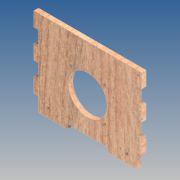
# Autodesk Inventor part: 2204_Housing Front_V1
Saved by Autodesk Inventor 2020 (Build 240168000, 168)
## iProperties
Created: 2019-11-08
Part Number: 2204_Housing Front_V1
Material: Wood (Birch)
Document SubType Name: Modeling
Designer: RFLab
Density: 0.55 g/cm^3
Appearance: Birch - Natural Polished
Author: RFLab
Autodesk Inventor part; units mm, degrees
ref_plane "YZ Plane" through (0, 0, 0) normal (1, 0, 0) x (0, 1, 0)
ref_plane "XZ Plane" through (0, 0, 0) normal (0, 1, 0) x (-1, 0, 0)
ref_plane "XY Plane" through (0, 0, 0) normal (0, 0, 1) x (1, 0, 0)
sketch "Sketch1" plane through (0, 0, 0) normal (0, 0, 1) x (1, 0, 0)
  line L0 (-75, 60) -> (75, 60)
  line L1 (75, 60) -> (75, -60)
  line L2 (75, -60) -> (-75, -60)
  line L3 (-75, -60) -> (-75, 60)
  point P0 (0, 0)
  dimension "d0" = 150
  dimension "d1" = 120
  dimension "d2" = 60
  dimension "d3" = 75
  constraints: 8 end point, 2 parallel, 1 horizontal, 1 perpendicular
  measures "d0" distance of L1.end L2.end
  measures "d1" distance of L0.end L1.end
  measures "d2" distance from line of point (0, 0) L2
  measures "d3" distance from line of L3 point (0, 0)
extrude "Extrusion1" add sketch "Sketch1" along normal blind 6.35
sketch "Sketch2" plane through (0, 0, 6.35) normal (0, 0, 1) x (1, 0, 0)
  line L0 (-75, 60) -> (-75, -60) projected
  line L1 (-75, 40) -> (-68.65, 40)
  line L2 (-68.65, 40) -> (-68.65, 20)
  line L3 (-68.65, 20) -> (-75, 20)
  line L4 (-75, 20) -> (-75, 40)
  line L5 (-75, 60) -> (-75, -60) projected
  line L6 (-75, 0) -> (-68.65, 0)
  line L7 (-68.65, 0) -> (-68.65, -20)
  line L8 (-68.65, -20) -> (-75, -20)
  line L9 (-75, -20) -> (-75, 0)
  line L10 (-75, -40) -> (-68.65, -40)
  line L11 (-68.65, -40) -> (-68.65, -60)
  line L12 (-68.65, -60) -> (-75, -60)
  line L13 (-75, -60) -> (-75, -40)
  line L14 (75, -60) -> (75, 60) projected
  line L15 (75, 40) -> (68.65, 40)
  line L16 (68.65, 40) -> (68.65, 20)
  line L17 (68.65, 20) -> (75, 20)
  line L18 (75, 20) -> (75, 40)
  line L19 (75, 0) -> (68.65, 0)
  line L20 (68.65, 0) -> (68.65, -20)
  line L21 (68.65, -20) -> (75, -20)
  line L22 (75, -20) -> (75, 0)
  line L23 (75, -40) -> (68.65, -40)
  line L24 (68.65, -40) -> (68.65, -60)
  line L25 (68.65, -60) -> (75, -60)
  line L26 (75, -60) -> (75, -40)
  line L27 (-75, -60) -> (75, -60) projected
  line L28 (-28.65, -60) -> (28.65, -60)
  line L29 (28.65, -60) -> (28.65, -53.65)
  line L30 (28.65, -53.65) -> (-28.65, -53.65)
  line L31 (-28.65, -53.65) -> (-28.65, -60)
  line L32 (75, 60) -> (-75, 60) projected
  line L33 (-28.65, 60) -> (28.65, 60)
  point P0 (0, 0)
  dimension "d6" = 6.35
  dimension "d7" = 20
  dimension "d8" = 20
  dimension "d9" = 20
  dimension "d10" = 20
  dimension "d11" = 20
  dimension "d12" = 20
  dimension "d13" = 20
  dimension "d22" = 57.3
  dimension "d23" = 46.35
  dimension "d24" = 46.35
  dimension "d26" = 6.35
  constraints: 58 end point, 14 parallel, 9 point on line, 8 horizontal, 7 equal length, 7 perpendicular, 2 midpoint
  measures "d6" distance of L1.start L1.end
  measures "d7" distance of L1.end L2.end
  measures "d8" distance of L1.start L0.start
  measures "d9" distance of L6.start L3.end
  measures "d10" distance of L10.start L8.end
  measures "d11" distance of L15.start L14.end
  measures "d12" distance of L19.start L17.end
  measures "d13" distance of L23.start L21.end
  measures "d22" distance of L29.end L30.end
  measures "d23" distance of L14.start L28.end
  measures "d24" distance of L14.end L33.end
  measures "d26" distance of L30.end L28.start
extrude "Extrusion2" cut sketch "Sketch2" against normal through all contours L1 L2 L3 L0 | L6 L7 L8 L0 | L14 L17 L16 L15 | L10 L11 L12 L0 | L14 L21 L20 L19 | L31 L30 L29 L27 | L14 L25 L24 L23
sketch "Sketch3" plane through (0, 0, 6.35) normal (0, 0, 1) x (1, 0, 0)
  circle A0 centre (0, -4.5) radius 27
  line L0 (-75, -60) -> (75, -60) projected
  line L1 (75, 40) -> (75, 60) projected
  point P0 (0, 0)
  dimension "d16" = 55.5
  dimension "d17" = 75
  dimension "d18" = 54
  constraints: 1 centre point
  measures "d16" distance from line of L0 A0.centre
  measures "d17" distance from line of L1 A0.centre
  measures "d18" diameter of A0
extrude "Extrusion3" cut sketch "Sketch3" against normal through all
sketch "Sketch4" plane through (0, 0, 6.35) normal (0, 0, 1) x (1, 0, 0)
  circle A0 centre (0, -4.5) radius 27 projected
  circle A1 centre (0, -4.5) radius 33.5
  circle A2 centre (23.6881, 19.1881) radius 1.75
  line L0 (0, -4.5) -> (33.5, -4.5)
  line L1 (0, -4.5) -> (23.6881, 19.1881)
  point P0 (0, 0)
  dimension "d27" = 67
  dimension "d28" = 45
  dimension "d29" = 3.5
  constraints: 4 end point, 2 centre point, 2 point on circle, 1 coincident, 1 horizontal
  measures "d27" diameter of A1
  measures "d28" angle of L1 L0
  measures "d29" diameter of A2
extrude "Extrusion4" cut sketch "Sketch4" against normal through all contours L1 A1 A2 | A2 A1 L1 | A1 A2
pattern_circular "Circular Pattern1" count 4 over 360 about axis through (0, -4.5, 6.35) along (0, 0, -1) of "Extrusion4"
sketch "Sketch5" plane through (0, 0, 6.35) normal (0, 0, 1) x (1, 0, 0)
  circle A0 centre (-54.9, -48) radius 1.75
  circle A1 centre (54.9, -48) radius 1.75
  line L0 (-68.65, -60) -> (-28.65, -60) projected
  line L1 (-75, -20) -> (-75, -40) projected
  line L2 (75, -40) -> (75, -20) projected
  line L3 (28.65, -60) -> (68.65, -60) projected
  point P0 (0, 0)
  dimension "d35" = 3.5
  dimension "d36" = 12
  dimension "d37" = 20.1
  dimension "d38" = 20.1
  dimension "d39" = 12
  constraints: 2 centre point, 1 equal radius
  measures "d35" diameter of A0
  measures "d36" distance from line of L0 A0.centre
  measures "d37" distance from line of L1 A0.centre
  measures "d38" distance from line of L2 A1.centre
  measures "d39" distance from line of L3 A1.centre
extrude "Extrusion5" cut sketch "Sketch5" against normal blind 10
equation "\"d2\" = 0.5 * d1"
equation "\"d3\" = 0.5 * d0"
equation "\"d11\" = d8"
equation "\"d12\" = d9"
equation "\"d13\" = d10"
equation "\"d22\" = d21"
equation "\"d24\" = d23"
equation "\"d26\" = d25"
equation "\"d21\" = 57.3"
equation "\"d25\" = 6.35"
body "Solid1"
